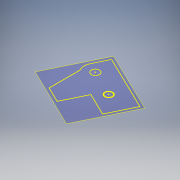
# Autodesk Inventor part: X-gan_holder
Saved by Autodesk Inventor 2016 SP2 (Build 200236200, 236)
## iProperties
Created: 2017-09-10
Part Number: X-gan_holder
Material: Generic
Document SubType Name: Sheet Metal
Designer: Admin
Density: 1 g/cm^3
Sheet Metal Rule: Default_mm
Appearance: Default
Author: Admin
Autodesk Inventor part; units mm, degrees
ref_plane "YZ Plane" through (0, 0, 0) normal (1, 0, 0) x (0, 1, 0)
ref_plane "XZ Plane" through (0, 0, 0) normal (0, 1, 0) x (-1, 0, 0)
ref_plane "XY Plane" through (0, 0, 0) normal (0, 0, 1) x (1, 0, 0)
ref_plane "Work Plane1" through (97.163, -47.1524, -1410) normal (0, 0, -1) x (-0.4365966, -0.8996574, 0)
sketch "Sketch1" plane through (97.163, -47.1524, -1410) normal (0, 0, -1) x (-0.4365966, -0.8996574, 0)
  circle A0 centre (0, 108) radius 15 projected
  circle A1 centre (-47.1524, 205.163) radius 13.2 projected
  line L0 (-83.4586, 176.9061) -> (-122.5647, 257.4887) projected
  line L1 (-122.5647, 257.4887) -> (16.8822, 325.1612) projected
  line L2 (16.8822, 325.1612) -> (117.2994, 118.24) projected
  line L3 (117.2994, 118.24) -> (18.3371, 70.2144) projected
  arc A2 (-21.7442, 72.0669) -> (18.3371, 70.2144) centre (0, 108) ccw projected
  line L4 (-21.7442, 72.0669) -> (-138.1767, 72.0669) projected
  line L5 (-138.1767, 72.0669) -> (-166.5555, 130.5446) projected
  line L6 (-166.5555, 130.5446) -> (-85.9729, 169.6507) projected
  circle A3 centre (-47.1524, 205.163) radius 15 projected
  circle A4 centre (0, 108) radius 15 projected
  line L7 (-21.7442, 72.0669) -> (-81.0881, 172.0213)
  arc A5 (-85.9729, 169.6507) -> (-83.4586, 176.9061) centre (-83.6554, 172.911) ccw projected
  point P0 (0, 108)
  constraints: 2 end point
extrude "Extrusion2" add sketch "Sketch1" along normal blind 15 contours L0 L1 L2 L3 A2 L7 A5 | L7 L4 L5 L6 A5
equation "\"BendRadius\" = Thickness"
equation "\"BendReliefWidth\" = Thickness"
equation "\"BendReliefDepth\" = 0.5 * Thickness"
equation "\"CornerReliefSize\" = 4 * Thickness"
equation "\"MinimumRemnant\" = 2 * Thickness"
equation "\"TransitionRadius\" = BendRadius"
equation "\"JacobiRadiusSize\" = BendRadius"
equation "\"GapSize\" = Thickness"
equation "\"Thickness\" = 0.5"
body "Solid2"
